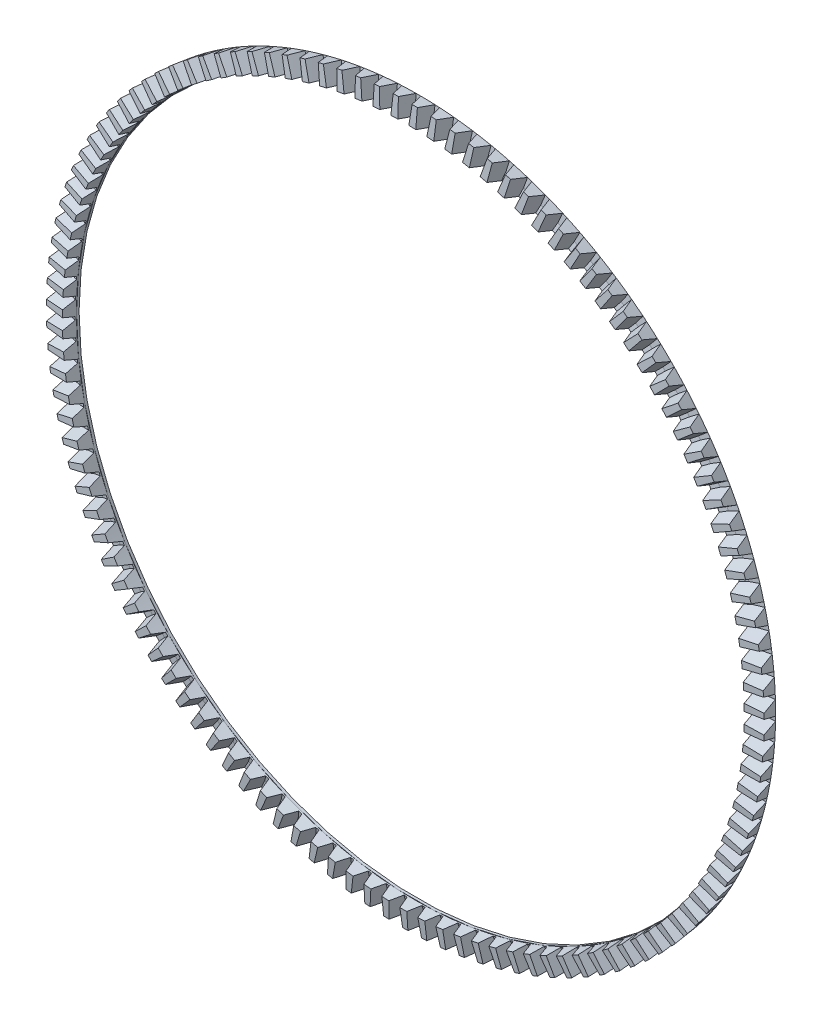
# Autodesk Inventor part: Bevel Gear1
Saved by Autodesk Inventor 2017 (Build 210142000, 142)
## iProperties
Created: 2017-01-10
Part Number: Bevel Gear1
Material: Steel, Mild
Document SubType Name: Modeling
Designer: David Kopala
Categories: <?xml version="1.0" encoding="UTF-16"?> <MemberInstance><Categories><FamilyTemplate><FamilyTemplateParameter ValueType="xs:double" Id="1" ObjectReferenceKey="da_z" ObjectType="kUserParameterObject"/><FamilyTemplateParameter ValueType="xs:double" Id="2" ObjectReferenceKey="da_b" ObjectType="kUserParameterObject"/><FamilyTemplateParameter ValueType="xs:double" Id="3" ObjectReferenceKey="da_beta" ObjectType="kUserParameterObject"/><FamilyTemplateParameter ValueType="xs:double" Id="4" ObjectReferenceKey="da_dae" ObjectType="kUserParameterObject"/><FamilyTemplateParameter ValueType="xs:double" Id="5" ObjectReferenceKey="da_ve" ObjectType="kUserParameterObject"/><FamilyTemplateParameter ValueType="xs:double" Id="6" ObjectReferenceKey="da_omega" ObjectType="kUserParameterObject"/><FamilyTemplateParameter ValueType="xs:string" Id="7" ObjectReferenceKey="EAIAABAAAAAAHwAAAAAAAIAAAAAAAAAA" ObjectType="83914240" SubObjectId="SurfaceGeometry"/></FamilyTemplate><ParamToTemplateMap><ParamToTemplate CategoryParameter="//CategoryParameter[@InternalName='046C89C9-8512-4d59-83FE-43B91F4F132A']" TemplateParameter="1"/><ParamToTemplate CategoryParameter="//CategoryParameter[@InternalName='2552DF32-E462-4b46-AEBF-C6C7768E72AC']" TemplateParameter="2"/><ParamToTemplate CategoryParameter="//CategoryParameter[@InternalName='C9EE641D-15FC-4fae-A226-E94C4372FDD7']" TemplateParameter="3"/><ParamToTemplate><ParamToTemplate CategoryParameter="//CategoryParameter[@InternalName='00B6519A-459B-49c7-AD84-2E56D39A5744']" ConstantValue="0.000000"/></ParamToTemplate><ParamToTemplate><ParamToTemplate CategoryParameter="//CategoryParameter[@InternalName='04B31F0E-C7A6-4894-AA32-9629BEFACF47']" ConstantValue="1.000000"/></ParamToTemplate><ParamToTemplate><ParamToTemplate CategoryParameter="//CategoryParameter[@InternalName='43CBEC2E-7847-49e7-A936-2F7889FCB2D9']" ConstantValue="0.200000"/></ParamToTemplate><ParamToTemplate><ParamToTemplate CategoryParameter="//CategoryParameter[@InternalName='B1EFC894-105D-4ebd-86BF-FA20ED196853']" ConstantValue="0.300000"/></ParamToTemplate><ParamToTemplate><ParamToTemplate CategoryParameter="//CategoryParameter[@InternalName='51175063-3D10-4879-93E8-6246FE8B403D']" ConstantValue="2061532430.657340"/></ParamToTemplate><ParamToTemplate><ParamToTemplate CategoryParameter="//CategoryParameter[@InternalName='A3A52E27-4454-46a9-B0BD-C932399B70AF']" ConstantValue="0.300000"/></ParamToTemplate><ParamToTemplate CategoryParameter="//CategoryParameter[@InternalName='2A200944-5A8C-41ca-B96E-8520D2E510F1']" TemplateParameter="4"/><ParamToTemplate><ParamToTemplate CategoryParameter="//CategoryParameter[@InternalName='1A637F62-92C8-44bc-B81F-10802510B579']" ConstantValue="28.774318"/></ParamToTemplate><ParamToTemplate CategoryParameter="//CategoryParameter[@InternalName='B52DD4BE-6863-48fb-BF58-89EF6F9EC65C']" TemplateParameter="5"/><ParamToTemplate><ParamToTemplate CategoryParameter="//CategoryParameter[@InternalName='3956BFF2-84D2-457d-93C2-9B0613DEBA67']" ConstantValue="1.570304"/></ParamToTemplate><ParamToTemplate CategoryParameter="//CategoryParameter[@InternalName='739CFA02-461B-4bf8-8049-181FCAD8B28F']" TemplateParameter="6"/><ParamToTemplate><ParamToTemplate CategoryParameter="//CategoryParameter[@InternalName='A27E999F-E2CE-4481-8A2A-EBF499C4C3C5']" ConstantValue="0.000000"/></ParamToTemplate><ParamToTemplate><ParamToTemplate CategoryParameter="//CategoryParameter[@InternalName='9E1B4470-B2D3-4ff1-B813-535BB4CDF51A']" ConstantValue="3523220.976809"/></ParamToTemplate><ParamToTemplate><ParamToTemplate CategoryParameter="//CategoryParameter[@InternalName='F8452263-BFF6-458c-9FB1-07C4B99E95CD']" ConstantValue="11397033.805607"/></ParamToTemplate><ParamToTemplate><ParamToTemplate CategoryParameter="//CategoryParameter[@InternalName='3E3BB259-FD49-497f-8171-6EBC954A3479']" ConstantValue="2.000000"/></ParamToTemplate><ParamToTemplate CategoryParameter="//CategoryParameter[@InternalName='27C3BAF2-7550-4e4b-AE2C-0DB134B7D9B7']" TemplateParameter="7"/></ParamToTemplateMap><Category DisplayName="Gear" InternalName="DC85795E-93AB-48d5-8EEE-5A27447B64BD" Mnemonic="Gear"><CategoryParameter DisplayName="z" InternalName="046C89C9-8512-4d59-83FE-43B91F4F132A" Mnemonic="z"/><CategoryParameter DisplayName="b" InternalName="2552DF32-E462-4b46-AEBF-C6C7768E72AC" Mnemonic="b"/><CategoryParameter DisplayName="||b|" InternalName="C9EE641D-15FC-4fae-A226-E94C4372FDD7" Mnemonic="beta"/><CategoryParameter DisplayName="x" InternalName="00B6519A-459B-49c7-AD84-2E56D39A5744" Mnemonic="x"/><CategoryParameter DisplayName="a*" InternalName="04B31F0E-C7A6-4894-AA32-9629BEFACF47" Mnemonic="a"/><CategoryParameter DisplayName="c*" InternalName="43CBEC2E-7847-49e7-A936-2F7889FCB2D9" Mnemonic="c"/><CategoryParameter DisplayName="r|.f|*" InternalName="B1EFC894-105D-4ebd-86BF-FA20ED196853" Mnemonic="rf"/><CategoryParameter DisplayName="E" InternalName="51175063-3D10-4879-93E8-6246FE8B403D" Mnemonic="E"/><CategoryParameter DisplayName="||m|" InternalName="A3A52E27-4454-46a9-B0BD-C932399B70AF" Mnemonic="mi"/><Category DisplayName="BevelGear" InternalName="0C98F69A-0C2B-4791-B2FE-7691BB227E77" Mnemonic="BevelGear"><CategoryParameter DisplayName="d|.ae|" InternalName="2A200944-5A8C-41ca-B96E-8520D2E510F1" Mnemonic="dae"/><CategoryParameter DisplayName="d|.ai|" InternalName="1A637F62-92C8-44bc-B81F-10802510B579" Mnemonic="dai"/><CategoryParameter DisplayName="A|.e|" InternalName="B52DD4BE-6863-48fb-BF58-89EF6F9EC65C" Mnemonic="ve"/><CategoryParameter DisplayName="A|.i|" InternalName="3956BFF2-84D2-457d-93C2-9B0613DEBA67" Mnemonic="vi"/><CategoryParameter DisplayName="||S|" InternalName="739CFA02-461B-4bf8-8049-181FCAD8B28F" Mnemonic="omega"/><CategoryParameter DisplayName="x|.t|" InternalName="A27E999F-E2CE-4481-8A2A-EBF499C4C3C5" Mnemonic="xt"/><CategoryParameter DisplayName="||s||.Flim|" InternalName="9E1B4470-B2D3-4ff1-B813-535BB4CDF51A" Mnemonic="sFlim"/><CategoryParameter DisplayName="||s||.Hlim|" InternalName="F8452263-BFF6-458c-9FB1-07C4B99E95CD" Mnemonic="sHlim"/><CategoryParameter DisplayName="type" InternalName="3E3BB259-FD49-497f-8171-6EBC954A3479" Mnemonic="type"/><CategoryParameter DisplayName="PitchDiameter" InternalName="27C3BAF2-7550-4e4b-AE2C-0DB134B7D9B7" Mnemonic="IDS_PITCHDIAM"/></Category></Category></Categories></MemberInstance>
Mass: 60.9118 g
Surface Area: 34.3074 cm^2
Volume: 7.7496 cm^3
Density: 7.86 g/cm^3
Appearance: Steel
Author: David Kopala
Autodesk Inventor part; units mm, degrees
ref_plane "Mesh Plane2" through (0, 0, 0) normal (0.9996515, 0.0263969, 0) x (0, 0, 1)
sketch "Teeth Body Sketch" plane through (0, 0, 0) normal (1, 0, 0) x (0, 1, 0)
  line L0 (0, 0) -> (150.7488, -22.0741) construction
  line L1 (150.7488, -22.0741) -> (151.4477, -16.5299)
  line L2 (151.4477, -16.5299) -> (0, 0) construction
  line L3 (151.13, -19.05) -> (0, 0) construction
  line L4 (143.2077, -20.9698) -> (143.8716, -15.703)
  line L5 (150.7488, -22.0741) -> (143.2077, -20.9698)
  line L6 (151.4477, -16.5299) -> (143.8716, -15.703)
  line L7 (0, -26.4884) -> (0, 4.4147) projected
  line L8 (0, -19.05) -> (151.4477, -19.05) construction
  dimension "d0" = 302.26
  dimension "d1" = 301.4976
  dimension "d2" = 302.8953
  dimension "d3" = 7.62
  dimension "d4" = 16.5299
  constraints: 16 end point, 4 point on line, 3 perpendicular, 2 collinear, 1 horizontal alignment, 1 vertical alignment
  measures "d0" diameter of L3.start L7
  measures "d1" diameter of L0.end L7
  measures "d2" diameter of L1.end L7
  measures "d3" distance between parallel lines of L1 L4
  measures "d4" vertical distance of L1.end L0.start
revolve "Teeth Body" add sketch "Teeth Body Sketch" angle 360 about axis through (0, 0, 0) along (0, 0, 1)
ref_plane "Tooth Plane" through (0, 151.13, -19.05) normal (0, -0.9921491, 0.1250608) x (1, 0, 0)
sketch "Start Sketch" plane through (0, 151.13, -19.05) normal (0, -0.9921491, 0.1250608) x (1, 0, 0)
  line L0 (0, -1426.9063) -> (0, 242.7392) projected
  arc A0 (-0.725, -3.7186) -> (-3.4821, 4.2114) centre (-393.3167, -135.7709) ccw
  arc A1 (3.4821, 4.2114) -> (0.725, -3.7186) centre (393.3167, -135.7709) ccw
  line L1 (-0.725, -3.7186) -> (0.725, -3.7186)
  arc A2 (3.4821, 4.2114) -> (-3.4821, 4.2114) centre (0, -1208.4521) ccw
  dimension "d7" = 414.2053
  dimension "d8" = 393.3167
  dimension "d9" = 1072.6812
  dimension "d57" = 1212.6685
  dimension "d58" = 1204.7336
  constraints: 6 point on circle, 3 centre point, 3 symmetric about line, 2 end point, 1 coincident, 1 perpendicular, 1 other
  measures "d7" radius of A0
  measures "d8" horizontal distance of point (0, -1208.452) A0.centre
  measures "d9" vertical distance of point (0, -1208.452) A0.centre
  measures "d57" radius of A2
  measures "d58" distance from line of A2.centre L1
sketch "End Sketch" plane through (0, 143.2926, -18.0621) normal (0, -0.9921491, 0.1250608) x (1, 0, 0)
  line L0 (0, -1352.5304) -> (0, 231.4772) projected
  arc A0 (-0.6882, -2.321) -> (-3.305, 5.2057) centre (-373.3132, -127.6574) ccw
  arc A1 (3.305, 5.2057) -> (0.6882, -2.321) centre (373.3132, -127.6574) ccw
  line L1 (-0.6882, -2.321) -> (0.6882, -2.321)
  arc A2 (3.305, 5.2057) -> (-3.305, 5.2057) centre (0, -1145.7836) ccw
  dimension "d12" = 393.1394
  dimension "d15" = 373.3132
  dimension "d16" = 1018.1262
  dimension "d59" = 1150.994
  dimension "d60" = 1143.4626
  constraints: 6 point on circle, 3 centre point, 3 symmetric about line, 2 end point, 1 coincident, 1 other
  measures "d12" radius of A0
  measures "d15" horizontal distance of A0.centre point (0, -1145.784)
  measures "d16" vertical distance of A0.centre point (0, -1145.784)
  measures "d59" radius of A2
  measures "d60" distance from line of A2.centre L1
loft "Loft" cut profiles "Start Sketch", "End Sketch"
pattern_circular "Circular Pattern" count 119 over 360 about axis through (0, 0, 0) along (0, 0, 1) of "Loft"
ref_plane "End Plane" through (0, 143.2926, -18.0621) normal (0, -0.9921491, 0.1250608) x (1, 0, 0)
sketch3d "3D Sketch Right"
ref_plane "End Plane Right" through (-2.8306, 143.2647, -18.0621) normal (0.0195986, -0.9919555, 0.1250608) x (0.9998049, 0.0197537, 0)
sketch "End Sketch Right" plane through (-2.8306, 143.2647, -18.0621) normal (0.0195986, -0.9919555, 0.1250608) x (0.9998049, 0.0197537, 0)
  arc A0 (-0.6882, -2.321) -> (-3.305, 5.2057) centre (-373.3132, -127.6574) ccw
  line L0 (0, -1378.5164) -> (0, 237.9232) projected
  arc A1 (3.305, 5.2057) -> (0.6882, -2.321) centre (373.3132, -127.6574) ccw
  line L1 (-0.6882, -2.321) -> (0.6882, -2.321)
  arc A2 (3.305, 5.2057) -> (-3.305, 5.2057) centre (0, -1145.7836) ccw
  dimension "d70" = 373.3132
  dimension "d71" = 1018.1262
  dimension "d72" = 393.1394
  dimension "d73" = 1143.4626
  dimension "d74" = 1150.994
  constraints: 6 point on circle, 3 centre point, 3 symmetric about line, 2 end point, 1 coincident, 1 perpendicular, 1 other
  measures "d70" horizontal distance of A2.centre A0.centre
  measures "d71" vertical distance of point (0, -1145.784) A0.centre
  measures "d72" radius of A0
  measures "d73" distance from line of point (0, -1145.784) L1
  measures "d74" radius of A2
feature "Loft Right" [suppressed]
pattern_circular "Circular Pattern Right" [suppressed]
sketch3d "3D Sketch Left"
ref_plane "End Plane Left" through (2.841, 143.2647, -18.0926) normal (-0.0196704, -0.9919279, 0.1252683) x (0.9998034, -0.0198266, 0)
sketch "End Sketch Left" plane through (2.841, 143.2647, -18.0926) normal (-0.0196704, -0.9919279, 0.1252683) x (0.9998034, -0.0198266, 0)
  line L0 (0, -1378.4997) -> (0, 237.967) projected
  arc A0 (-0.6882, -2.2908) -> (-3.305, 5.2359) centre (-373.3132, -127.6271) ccw
  arc A1 (3.305, 5.2359) -> (0.6882, -2.2908) centre (373.3132, -127.6271) ccw
  line L1 (-0.6882, -2.2908) -> (0.6882, -2.2908)
  ellipse E0 centre (0, -15.5793) end of major axis (143.8716, -15.5793) minor radius 18.0225 projected
  arc A2 (3.305, 5.2359) -> (-3.305, 5.2359) centre (0, -1145.7533) ccw
  dimension "d56" = 18.0225
  dimension "d30" = 393.1394
  dimension "d31" = 373.3132
  dimension "d32" = 1018.1262
  dimension "d61" = 1150.994
  dimension "d62" = 1143.4626
  constraints: 6 point on circle, 3 centre point, 3 symmetric about line, 2 end point, 1 coincident, 2 other
  measures "d30" radius of A0
  measures "d31" horizontal distance of point (0, -1145.753) A0.centre
  measures "d32" vertical distance of A0.centre point (0, -1145.753)
  measures "d61" radius of A2
  measures "d62" distance from line of point (0, -1145.753) L1
feature "Loft Left" [suppressed]
pattern_circular "Circular Pattern Left" [suppressed]
sketch "Body Sketch" plane through (0, 0, 0) normal (1, 0, 0) x (0, 1, 0)
  line L0 (0, -22.2964) -> (0, -20.7376) projected
  line L1 (150.7488, -22.0741) -> (143.2077, -20.9698) projected
  line L2 (143.2077, -20.9698) -> (0, -20.9698)
  line L3 (150.7488, -22.0741) -> (0, -22.0741)
  constraints: 4 end point, 2 perpendicular, 2 point on line
revolve "Fix Body" add sketch "Body Sketch" angle 360 about axis through (0, 0, 0) along (0, 0, 1)
sketch "Sketch6" plane through (0, 0, 0) normal (1, 0, 0) x (0, 1, 0)
  line L0 (151.13, -19.05) -> (0, 0) projected
  line L1 (0, -22.86) -> (0, 3.81) projected
surface revolve "Pitch Diameter" sketch "Sketch6" angle 360 about axis through (0, 0, 0) along (0, 0, 1) shown no curves L0
sketch "Sketch8" plane through (0, 0, -20.9698) normal (0, 0, 1) x (1, 0, 0)
  circle A0 centre (0, 0) radius 143.2052
  dimension "d92" = 286.4104
  constraints: 1 centre point, 1 coincident
  measures "d92" diameter of A0
extrude "Extrusion1" cut sketch "Sketch8" against normal blind 25.4
equation "\"d0\" = da_de"
equation "\"d1\" = da_dfe"
equation "\"d2\" = da_dae"
equation "\"d3\" = da_b"
equation "\"d4\" = da_ve"
equation "\"d7\" = fd_rr"
equation "\"d8\" = fd_x"
equation "\"d9\" = fd_y"
equation "\"d57\" = 0.5 * fd_dva + 0.3 * da_he"
equation "\"d58\" = 0.5 * fd_dva - 1.12 * da_he"
equation "\"da_teethtype\" = 0"
equation "\"da_b\" = 7.62"
equation "\"da_de\" = 302.26"
equation "\"da_dae\" = 302.89531"
equation "\"da_dfe\" = 301.49763"
equation "\"da_le\" = 152.3259"
equation "\"da_omega\" = 90deg"
equation "\"da_beta\" = 0"
equation "\"da_delta\" = 82.815733deg"
equation "\"da_alpha\" = 20deg"
equation "\"da_he\" = 5.588"
equation "\"da_ve\" = 16.52994"
equation "\"da_zv\" = 951.53711"
equation "\"fd_loft\" = da_b + 0.05 * da_he"
equation "\"fd_x\" = fd_x1 + fd_x2"
equation "\"fd_y\" = fd_y1 - fd_y2"
equation "\"fd_dd\" = fd_dva - 0.8 * da_he"
equation "\"da_dvw\" = 2416.90426"
equation "\"d11\" = fd_loft"
equation "\"da_dm\" = 294.69982"
equation "\"da_x\" = 0"
equation "\"da_m\" = 2.54"
equation "\"d50\" = da_omega"
equation "\"fd_rr\" = 414.205299"
equation "\"fd_dva\" = 2421.984259"
equation "\"fd_x1\" = 1.99491"
equation "\"fd_x2\" = 391.321779"
equation "\"fd_y1\" = 1208.450483"
equation "\"fd_y2\" = 135.769272"
body "Solid1"
body "Srf1"
